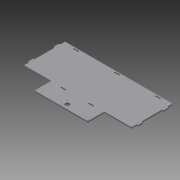
# Autodesk Inventor part: FRAME BOTTOM
Saved by Autodesk Inventor 2013 (Build 170138000, 138)
## iProperties
Created: 2014-03-04
Part Number: FRAME BOTTOM
Material: Generic
Document SubType Name: Modeling
Designer: employee
Density: 1 g/cm^3
Author: employee
Autodesk Inventor part; units mm, degrees
ref_plane "YZ Plane" through (0, 0, 0) normal (1, 0, 0) x (0, 1, 0)
ref_plane "XZ Plane" through (0, 0, 0) normal (0, 1, 0) x (-1, 0, 0)
ref_plane "XY Plane" through (0, 0, 0) normal (0, 0, 1) x (1, 0, 0)
sketch "Sketch1" plane through (0, 0, 0) normal (0, 0, 1) x (1, 0, 0)
  line L0 (-130, -81.477) -> (130, -81.477)
  line L1 (130, -81.477) -> (130, 0)
  line L2 (130, 0) -> (-130, 0)
  line L3 (-130, 0) -> (-130, -81.477)
  line L4 (262.5, 0) -> (-262.5, 0)
  line L5 (-262.5, 0) -> (-262.5, 200)
  line L6 (-262.5, 200) -> (262.5, 200)
  line L7 (262.5, 200) -> (262.5, 0)
  point P0 (0, 0)
  point P1 (0, 0)
  dimension "d0" = 260
  dimension "d2" = 81.477
  dimension "d3" = 525
  dimension "d4" = 200
  constraints: 16 end point, 4 parallel, 2 coincident, 2 horizontal, 2 midpoint, 2 perpendicular
  measures "d0" distance of L1.end L2.end
  measures "d2" distance of L0.end L1.end
  measures "d3" distance of L5.end L6.end
  measures "d4" distance of L4.end L5.end
extrude "Extrusion1" add sketch "Sketch1" along normal blind 6.477
fillet "Fillet1" radius 5 2 edges at (-130, -81.477, 3.2385) (130, -81.477, 3.2385)
sketch "Sketch2" plane through (0, 0, 0) normal (0, 0, -1) x (-1, 0, 0)
  line L0 (-111.6967, -32.977) -> (-111.6967, -8.977) projected
  line L1 (-111.6967, -8.977) -> (-122.3033, -8.977) projected
  line L2 (-122.3033, -8.977) -> (-122.3033, -32.977) projected
  line L3 (-122.3033, -32.977) -> (-111.6967, -32.977) projected
  arc A0 (-109, -81.477) -> (-104, -76.477) centre (-109, -76.477) ccw projected
  line L4 (-109, -81.477) -> (-125, -81.477) projected
  arc A1 (-130, -76.477) -> (-125, -81.477) centre (-125, -76.477) ccw projected
  line L5 (-130, -76.477) -> (-130, -11.477) projected
  arc A2 (-125, -6.477) -> (-130, -11.477) centre (-125, -11.477) ccw projected
  line L6 (-125, -6.477) -> (-109, -6.477) projected
  arc A3 (-104, -11.477) -> (-109, -6.477) centre (-109, -11.477) ccw projected
  line L7 (-104, -11.477) -> (-104, -76.477) projected
  line L8 (-111.6967, -54.977) -> (-122.3033, -54.977) projected
  line L9 (-122.3033, -54.977) -> (-122.3033, -78.977) projected
  line L10 (-122.3033, -78.977) -> (-111.6967, -78.977) projected
  line L11 (-111.6967, -78.977) -> (-111.6967, -54.977) projected
  line L12 (-108, -29.977) -> (-108, -25.977) projected
  line L13 (-108, -25.977) -> (-109.5, -25.977) projected
  line L14 (-109.5, -25.977) -> (-109.5, -29.977) projected
  line L15 (-109.5, -29.977) -> (-108, -29.977) projected
  line L16 (-124.5, -29.977) -> (-124.5, -25.977) projected
  line L17 (-124.5, -25.977) -> (-126, -25.977) projected
  line L18 (-126, -25.977) -> (-126, -29.977) projected
  line L19 (-126, -29.977) -> (-124.5, -29.977) projected
  line L20 (-109.5, -11.977) -> (-109.5, -15.977) projected
  line L21 (-109.5, -15.977) -> (-108, -15.977) projected
  line L22 (-108, -15.977) -> (-108, -11.977) projected
  line L23 (-108, -11.977) -> (-109.5, -11.977) projected
  line L24 (-126, -11.977) -> (-126, -15.977) projected
  line L25 (-126, -15.977) -> (-124.5, -15.977) projected
  line L26 (-124.5, -15.977) -> (-124.5, -11.977) projected
  line L27 (-124.5, -11.977) -> (-126, -11.977) projected
  line L28 (-124.5, -75.977) -> (-124.5, -71.977) projected
  line L29 (-124.5, -71.977) -> (-126, -71.977) projected
  line L30 (-126, -71.977) -> (-126, -75.977) projected
  line L31 (-126, -75.977) -> (-124.5, -75.977) projected
  line L32 (-108, -57.977) -> (-109.5, -57.977) projected
  line L33 (-109.5, -57.977) -> (-109.5, -61.977) projected
  line L34 (-109.5, -61.977) -> (-108, -61.977) projected
  line L35 (-108, -61.977) -> (-108, -57.977) projected
  line L36 (-126, -57.977) -> (-126, -61.977) projected
  line L37 (-126, -61.977) -> (-124.5, -61.977) projected
  line L38 (-124.5, -61.977) -> (-124.5, -57.977) projected
  line L39 (-124.5, -57.977) -> (-126, -57.977) projected
  line L40 (-109.5, -75.977) -> (-108, -75.977) projected
  line L41 (-108, -75.977) -> (-108, -71.977) projected
  line L42 (-108, -71.977) -> (-109.5, -71.977) projected
  line L43 (-109.5, -71.977) -> (-109.5, -75.977) projected
  line L44 (122.3033, -32.977) -> (122.3033, -8.977) projected
  line L45 (122.3033, -8.977) -> (111.6967, -8.977) projected
  line L46 (111.6967, -8.977) -> (111.6967, -32.977) projected
  line L47 (111.6967, -32.977) -> (122.3033, -32.977) projected
  arc A4 (125, -81.477) -> (130, -76.477) centre (125, -76.477) ccw projected
  line L48 (125, -81.477) -> (109, -81.477) projected
  arc A5 (104, -76.477) -> (109, -81.477) centre (109, -76.477) ccw projected
  line L49 (104, -76.477) -> (104, -11.477) projected
  arc A6 (109, -6.477) -> (104, -11.477) centre (109, -11.477) ccw projected
  line L50 (109, -6.477) -> (125, -6.477) projected
  arc A7 (130, -11.477) -> (125, -6.477) centre (125, -11.477) ccw projected
  line L51 (130, -11.477) -> (130, -76.477) projected
  line L52 (122.3033, -54.977) -> (111.6967, -54.977) projected
  line L53 (111.6967, -54.977) -> (111.6967, -78.977) projected
  line L54 (111.6967, -78.977) -> (122.3033, -78.977) projected
  line L55 (122.3033, -78.977) -> (122.3033, -54.977) projected
  line L56 (126, -29.977) -> (126, -25.977) projected
  line L57 (126, -25.977) -> (124.5, -25.977) projected
  line L58 (124.5, -25.977) -> (124.5, -29.977) projected
  line L59 (124.5, -29.977) -> (126, -29.977) projected
  line L60 (109.5, -29.977) -> (109.5, -25.977) projected
  line L61 (109.5, -25.977) -> (108, -25.977) projected
  line L62 (108, -25.977) -> (108, -29.977) projected
  line L63 (108, -29.977) -> (109.5, -29.977) projected
  line L64 (124.5, -11.977) -> (124.5, -15.977) projected
  line L65 (124.5, -15.977) -> (126, -15.977) projected
  line L66 (126, -15.977) -> (126, -11.977) projected
  line L67 (126, -11.977) -> (124.5, -11.977) projected
  line L68 (108, -11.977) -> (108, -15.977) projected
  line L69 (108, -15.977) -> (109.5, -15.977) projected
  line L70 (109.5, -15.977) -> (109.5, -11.977) projected
  line L71 (109.5, -11.977) -> (108, -11.977) projected
  line L72 (109.5, -75.977) -> (109.5, -71.977) projected
  line L73 (109.5, -71.977) -> (108, -71.977) projected
  line L74 (108, -71.977) -> (108, -75.977) projected
  line L75 (108, -75.977) -> (109.5, -75.977) projected
  line L76 (126, -57.977) -> (124.5, -57.977) projected
  line L77 (124.5, -57.977) -> (124.5, -61.977) projected
  line L78 (124.5, -61.977) -> (126, -61.977) projected
  line L79 (126, -61.977) -> (126, -57.977) projected
  line L80 (108, -57.977) -> (108, -61.977) projected
  line L81 (108, -61.977) -> (109.5, -61.977) projected
  line L82 (109.5, -61.977) -> (109.5, -57.977) projected
  line L83 (109.5, -57.977) -> (108, -57.977) projected
  line L84 (124.5, -75.977) -> (126, -75.977) projected
  line L85 (126, -75.977) -> (126, -71.977) projected
  line L86 (126, -71.977) -> (124.5, -71.977) projected
  line L87 (124.5, -71.977) -> (124.5, -75.977) projected
  point P0 (0, 0)
extrude "Extrusion2" cut sketch "Sketch2" against normal through all contours L15 L14 L13 L12 | L19 L18 L17 L16 | L23 L22 L21 L20 | L27 L26 L25 L24 | L31 L30 L29 L28 | L35 L34 L33 L32 | L39 L38 L37 L36 | L43 L42 L41 L40 | L59 L58 L57 L56 | L63 L62 L61 L60 | L67 L66 L65 L64 | L71 L70 L69 L68 | L75 L74 L73 L72 | L79 L78 L77 L76 | L83 L82 L81 L80 | L87 L86 L85 L84
sketch "Sketch3" plane through (0, 0, 0) normal (0, 0, -1) x (-1, 0, 0)
  line L0 (125, -81.477) -> (-125, -81.477) projected
  line L1 (11.5, -81.477) -> (-30.5, -81.477)
  line L2 (-30.5, -81.477) -> (-30.5, -39.477)
  line L3 (-30.5, -39.477) -> (11.5, -39.477)
  line L4 (11.5, -39.477) -> (11.5, -81.477)
  circle A0 centre (-9.5, -60.477) radius 11
  line L5 (-25, -44.977) -> (6, -44.977)
  line L6 (6, -44.977) -> (6, -75.977)
  line L7 (6, -75.977) -> (-25, -75.977)
  line L8 (-25, -75.977) -> (-25, -44.977)
  circle A1 centre (-25, -75.977) radius 1.5
  circle A2 centre (6, -75.977) radius 1.5
  circle A3 centre (6, -44.977) radius 1.5
  circle A4 centre (-25, -44.977) radius 1.5
  point P0 (0, 0)
  point P1 (-9.5, -39.477)
  point P2 (11.5, -60.477)
  dimension "d10" = 9.5
  dimension "d11" = 42
  dimension "d12" = 22
  dimension "d13" = 31
  dimension "d14" = 3
  constraints: 16 end point, 5 centre point, 5 coincident, 3 equal radius, 2 horizontal, 2 midpoint, 2 parallel, 2 perpendicular, 1 horizontal alignment, 1 point on line, 1 vertical alignment, 9 other
  measures "d10" horizontal distance of point (0, 0) point (-9.5, -39.477)
  measures "d11" distance of L3.end L1.start
  measures "d12" diameter of A0
  measures "d13" distance of L6.end L7.end
  measures "d14" diameter of A1
extrude "Extrusion3" cut sketch "Sketch3" against normal through all contours A0 | L8 A4 L5 | L5 A4 L8 | A3 L6 L5 | L5 L6 A3 | A1 L7 L8 | L8 L7 A1 | A2 L7 L6 | L6 L7 A2
sketch "Sketch4" plane through (0, 0, 6.477) normal (0, 0, 1) x (1, 0, 0)
  line L0 (262.5, 200) -> (-262.5, 200) projected
  line L1 (-262.5, 200) -> (-262.5, 0) projected
  line L2 (-262.5, 0) -> (-130, 0) projected
  line L3 (-208.75, 0) -> (-183.75, 0)
  line L4 (-183.75, 0) -> (-183.75, -6.477)
  line L5 (-183.75, -6.477) -> (-208.75, -6.477)
  line L6 (-208.75, -6.477) -> (-208.75, 0)
  line L7 (-262.5, 25) -> (-268.977, 25)
  line L8 (-268.977, 25) -> (-268.977, 50)
  line L9 (-268.977, 50) -> (-262.5, 50)
  line L10 (-262.5, 50) -> (-262.5, 25)
  line L11 (-262.5, 175) -> (-268.977, 175)
  line L12 (-268.977, 175) -> (-268.977, 150)
  line L13 (-268.977, 150) -> (-262.5, 150)
  line L14 (-262.5, 150) -> (-262.5, 175)
  point P0 (0, 0)
  point P1 (-196.25, 0)
  point P2 (-196.25, 0)
  dimension "d17" = 25
  dimension "d18" = 25
  dimension "d19" = 25
  dimension "d20" = 6.477
  constraints: 24 end point, 6 parallel, 4 equal length, 3 horizontal, 3 perpendicular, 3 point on line, 2 midpoint, 1 coincident
  measures "d17" distance between parallel lines of L7 L2
  measures "d18" distance between parallel lines of L0 L11
  measures "d19" distance of L4.end L5.end
  measures "d20" distance of L5.end L3.start
extrude "Extrusion4" add sketch "Sketch4" against normal up to surface (6.477 mm away) contours L1 L7 L8 L9 | L1 L13 L12 L11
sketch "Sketch5" plane through (0, 0, 6.477) normal (0, 0, 1) x (1, 0, 0)
  line L0 (-268.977, 175) -> (-268.977, 150) projected
  line L1 (-268.977, 50) -> (-268.977, 25) projected
  line L2 (-260, 164.5) -> (-258.5, 164.5)
  line L3 (-258.5, 164.5) -> (-258.5, 160.5)
  line L4 (-258.5, 160.5) -> (-260, 160.5)
  line L5 (-260, 160.5) -> (-260, 164.5)
  line L6 (-260, 39.5) -> (-258.5, 39.5)
  line L7 (-258.5, 39.5) -> (-258.5, 35.5)
  line L8 (-258.5, 35.5) -> (-260, 35.5)
  line L9 (-260, 35.5) -> (-260, 39.5)
  point P0 (-262.5, 150)
  point P1 (0, 0)
  point P2 (-268.977, 37.5)
  point P3 (-260, 37.5)
  point P4 (-268.977, 162.5)
  point P5 (-260, 162.5)
  dimension "d23" = 2.5
  dimension "d24" = 4
  dimension "d25" = 1.5
  constraints: 16 end point, 4 midpoint, 4 parallel, 2 equal length, 2 horizontal, 2 horizontal alignment, 2 perpendicular, 1 vertical alignment
  measures "d23" horizontal distance of L4.end point (-262.5, 150)
  measures "d24" distance of L2.end L3.end
  measures "d25" distance of L2.start L2.end
extrude "Extrusion5" cut sketch "Sketch5" against normal through all
mirror "Mirror2" about plane through (0, 0, 0) normal (1, 0, 0) of "Extrusion4", "Extrusion5"
sketch "Sketch6" plane through (0, 0, 6.477) normal (0, 0, 1) x (1, 0, 0)
  line L0 (-187.5, 195) -> (-212.5, 195) projected
  line L1 (-187.5, 195) -> (-212.5, 195) projected
  line L2 (-212.5, 195) -> (-212.5, 188.523) projected
  line L3 (-187.5, 188.523) -> (-212.5, 188.523) projected
  line L4 (-187.5, 195) -> (-187.5, 188.523) projected
  line L5 (12.5, 195) -> (-12.5, 195) projected
  line L6 (-12.5, 195) -> (-12.5, 188.523) projected
  line L7 (12.5, 188.523) -> (-12.5, 188.523) projected
  line L8 (12.5, 195) -> (12.5, 188.523) projected
  line L9 (187.5, 195) -> (212.5, 195) projected
  line L10 (187.5, 195) -> (187.5, 188.523) projected
  line L11 (187.5, 188.523) -> (212.5, 188.523) projected
  line L12 (212.5, 195) -> (212.5, 188.523) projected
  line L13 (80, 0) -> (55, 0) projected
  line L14 (55, -6.477) -> (55, 0) projected
  line L15 (55, -6.477) -> (80, -6.477) projected
  line L16 (80, -6.477) -> (80, 0) projected
  line L17 (-80, 0) -> (-55, 0) projected
  line L18 (-80, -6.477) -> (-80, 0) projected
  line L19 (-55, -6.477) -> (-80, -6.477) projected
  line L20 (-55, -6.477) -> (-55, 0) projected
  point P0 (0, 0)
extrude "Extrusion6" cut sketch "Sketch6" against normal through all
sketch "Sketch7" plane through (0, 0, 6.477) normal (0, 0, 1) x (1, 0, 0)
  line L0 (-22.977, -71.477) -> (-22.977, -51.477) projected
  line L1 (-16.5, -71.477) -> (-22.977, -71.477) projected
  line L2 (-16.5, -51.477) -> (-16.5, -71.477) projected
  line L3 (-16.5, -51.477) -> (-22.977, -51.477) projected
  line L4 (35.5, -71.477) -> (35.5, -51.477) projected
  line L5 (41.977, -71.477) -> (35.5, -71.477) projected
  line L6 (41.977, -51.477) -> (41.977, -71.477) projected
  line L7 (41.977, -51.477) -> (35.5, -51.477) projected
  point P0 (0, 0)
extrude "Extrusion7" cut sketch "Sketch7" against normal through all
sketch "Sketch8" plane through (0, 0, 6.477) normal (0, 0, 1) x (1, 0, 0)
  line L0 (-22.977, -71.477) -> (-22.977, -51.477) projected
  line L1 (-22.977, -51.477) -> (-16.5, -51.477) projected
  line L2 (-80, -6.477) -> (-80, 0) projected
  line L3 (-80, 0) -> (-55, 0) projected
  line L4 (-55, -6.477) -> (-80, -6.477) projected
  line L5 (-26.977, -59.477) -> (-25.477, -59.477)
  line L6 (-25.477, -59.477) -> (-25.477, -63.477)
  line L7 (-25.477, -63.477) -> (-26.977, -63.477)
  line L8 (-26.977, -63.477) -> (-26.977, -59.477)
  line L9 (-25.477, -63.477) -> (-14, -63.477)
  line L10 (-14, -63.477) -> (-14, -59.477)
  line L11 (-14, -59.477) -> (-25.477, -59.477)
  line L12 (-25.477, -59.477) -> (-25.477, -63.477)
  line L13 (-14, -59.477) -> (-12.5, -59.477)
  line L14 (-12.5, -59.477) -> (-12.5, -63.477)
  line L15 (-12.5, -63.477) -> (-14, -63.477)
  line L16 (-14, -63.477) -> (-14, -59.477)
  line L17 (31.5, -59.477) -> (33, -59.477)
  line L18 (33, -59.477) -> (33, -63.477)
  line L19 (33, -63.477) -> (31.5, -63.477)
  line L20 (31.5, -63.477) -> (31.5, -59.477)
  line L21 (33, -63.477) -> (44.477, -63.477)
  line L22 (44.477, -63.477) -> (44.477, -59.477)
  line L23 (44.477, -59.477) -> (33, -59.477)
  line L24 (33, -59.477) -> (33, -63.477)
  line L25 (44.477, -59.477) -> (45.977, -59.477)
  line L26 (45.977, -59.477) -> (45.977, -63.477)
  line L27 (45.977, -63.477) -> (44.477, -63.477)
  line L28 (44.477, -63.477) -> (44.477, -59.477)
  line L29 (-69.5, 2.5) -> (-65.5, 2.5)
  line L30 (-65.5, 2.5) -> (-65.5, -8.977) construction
  line L31 (-65.5, -8.977) -> (-69.5, -8.977)
  line L32 (-69.5, -8.977) -> (-69.5, 2.5)
  line L33 (-69.5, -8.977) -> (-65.5, -8.977)
  line L34 (-65.5, -8.977) -> (-65.5, -10.477)
  line L35 (-65.5, -10.477) -> (-69.5, -10.477)
  line L36 (-69.5, -10.477) -> (-69.5, -8.977)
  line L37 (-69.5, 2.5) -> (-65.5, 2.5)
  line L38 (-65.5, 2.5) -> (-65.5, 4)
  line L39 (-65.5, 4) -> (-69.5, 4)
  line L40 (-69.5, 4) -> (-69.5, 2.5)
  line L41 (65.5, 2.5) -> (69.5, 2.5)
  line L42 (69.5, 2.5) -> (69.5, -8.977) construction
  line L43 (69.5, -8.977) -> (65.5, -8.977)
  line L44 (65.5, -8.977) -> (65.5, 2.5)
  line L45 (65.5, -8.977) -> (69.5, -8.977)
  line L46 (69.5, -8.977) -> (69.5, -10.477)
  line L47 (69.5, -10.477) -> (65.5, -10.477)
  line L48 (65.5, -10.477) -> (65.5, -8.977)
  line L49 (65.5, 2.5) -> (69.5, 2.5)
  line L50 (69.5, 2.5) -> (69.5, 4)
  line L51 (69.5, 4) -> (65.5, 4)
  line L52 (65.5, 4) -> (65.5, 2.5)
  line L53 (198, 197.5) -> (202, 197.5)
  line L54 (202, 197.5) -> (202, 186.023) construction
  line L55 (202, 186.023) -> (198, 186.023)
  line L56 (198, 186.023) -> (198, 197.5)
  line L57 (198, 186.023) -> (202, 186.023)
  line L58 (202, 186.023) -> (202, 184.523)
  line L59 (202, 184.523) -> (198, 184.523)
  line L60 (198, 184.523) -> (198, 186.023)
  line L61 (198, 197.5) -> (202, 197.5)
  line L62 (202, 197.5) -> (202, 199)
  line L63 (202, 199) -> (198, 199)
  line L64 (198, 199) -> (198, 197.5)
  line L65 (-2, 197.5) -> (2, 197.5)
  line L66 (2, 197.5) -> (2, 186.023) construction
  line L67 (2, 186.023) -> (-2, 186.023)
  line L68 (-2, 186.023) -> (-2, 197.5)
  line L69 (-2, 186.023) -> (2, 186.023)
  line L70 (2, 186.023) -> (2, 184.523)
  line L71 (2, 184.523) -> (-2, 184.523)
  line L72 (-2, 184.523) -> (-2, 186.023)
  line L73 (-2, 197.5) -> (2, 197.5)
  line L74 (2, 197.5) -> (2, 199)
  line L75 (2, 199) -> (-2, 199)
  line L76 (-2, 199) -> (-2, 197.5)
  line L77 (-202, 197.5) -> (-198, 197.5)
  line L78 (-198, 197.5) -> (-198, 186.023) construction
  line L79 (-198, 186.023) -> (-202, 186.023)
  line L80 (-202, 186.023) -> (-202, 197.5)
  line L81 (-202, 186.023) -> (-198, 186.023)
  line L82 (-198, 186.023) -> (-198, 184.523)
  line L83 (-198, 184.523) -> (-202, 184.523)
  line L84 (-202, 184.523) -> (-202, 186.023)
  line L85 (-202, 197.5) -> (-198, 197.5)
  line L86 (-198, 197.5) -> (-198, 199)
  line L87 (-198, 199) -> (-202, 199)
  line L88 (-202, 199) -> (-202, 197.5)
  point P0 (0, 0)
  point P1 (-19.7385, -59.477)
  point P2 (-19.7385, -51.477)
  point P3 (-25.477, -61.477)
  point P4 (-22.977, -61.477)
  point P5 (38.7385, -59.477)
  point P6 (33, -61.477)
  point P7 (35.5, -61.477)
  point P8 (-67.5, 2.5)
  point P9 (-67.5, 0)
  point P10 (-80, -3.2385)
  point P11 (-69.5, -3.2385)
  point P12 (67.5, 2.5)
  point P13 (67.5, 0)
  point P14 (65.5, -3.2385)
  point P15 (200, 197.5)
  point P16 (200, 195)
  point P17 (198, 191.7615)
  point P18 (0, 197.5)
  point P19 (0, 195)
  point P20 (-2, 191.7615)
  point P21 (-200, 197.5)
  point P22 (-200, 195)
  point P23 (-202, 191.7615)
  dimension "d33" = 2.5
  dimension "d34" = 1.5
  dimension "d35" = 4
  dimension "d36" = 1.5
  dimension "d37" = 4
  dimension "d38" = 2.5
  dimension "d39" = 1.5
  dimension "d40" = 4
  dimension "d41" = 1.5
  dimension "d42" = 4
  dimension "d43" = 1.5
  dimension "d44" = 4
  dimension "d45" = 1.5
  dimension "d46" = 4
  dimension "d47" = 1.5
  dimension "d48" = 4
  constraints: 168 end point, 42 parallel, 21 horizontal, 21 perpendicular, 18 midpoint, 11 vertical alignment, 7 collinear, 5 coincident, 5 horizontal alignment
  measures "d33" distance between parallel lines of L0 L12
  measures "d34" distance of L6.end L7.end
  measures "d35" distance of L7.end L5.start
  measures "d36" distance of L21.start L19.end
  measures "d37" distance of L19.end L17.start
  measures "d38" distance from line of L4 L31.end
  measures "d39" distance of L33.end L34.end
  measures "d40" distance of L34.end L35.end
  measures "d41" distance of L45.end L47.start
  measures "d42" distance of L47.start L48.start
  measures "d43" distance of L57.end L59.start
  measures "d44" distance of L59.start L60.start
  measures "d45" distance of L69.end L71.start
  measures "d46" distance of L71.start L72.start
  measures "d47" distance of L81.end L83.start
  measures "d48" distance of L83.start L84.start
extrude "Extrusion8" cut sketch "Sketch8" against normal through all contours L7 L8 L5 L6 | L10 L13 L14 L15 | L40 L39 L38 L29 | L31 L34 L35 L36 | L17 L18 L19 L20 | L25 L26 L27 L22 | L52 L51 L50 L41 | L43 L46 L47 L48 | L64 L63 L62 L53 | L55 L58 L59 L60 | L76 L75 L74 L65 | L67 L70 L71 L72 | L88 L87 L86 L77 | L79 L82 L83 L84
sketch "Sketch9" plane through (0, 0, 6.477) normal (0, 0, 1) x (1, 0, 0)
  circle A0 centre (9.5, -60.477) radius 11 projected
  line L0 (5.5, -31.477) -> (7, -31.477)
  line L1 (7, -31.477) -> (7, -35.477)
  line L2 (7, -35.477) -> (5.5, -35.477)
  line L3 (5.5, -35.477) -> (5.5, -31.477)
  line L4 (13.5, -31.477) -> (12, -31.477)
  line L5 (12, -31.477) -> (12, -35.477)
  line L6 (12, -35.477) -> (13.5, -35.477)
  line L7 (13.5, -35.477) -> (13.5, -31.477)
  line L8 (7, -35.477) -> (12, -35.477)
  point P0 (0, 0)
  point P1 (9.5, -35.477)
  dimension "d51" = 2.5
  dimension "d52" = 1.5
  dimension "d53" = 4
  dimension "d54" = 25
  constraints: 18 end point, 4 parallel, 3 horizontal, 2 equal length, 2 perpendicular, 1 midpoint, 1 vertical alignment
  measures "d51" horizontal distance of L1.end A0.centre
  measures "d52" distance of L4.start L4.end
  measures "d53" distance of L6.end L4.start
  measures "d54" distance from line of A0.centre L8
extrude "Extrusion9" cut sketch "Sketch9" against normal through all contours L5 L4 L7 L6 | L0 L1 L2 L3
sketch "Sketch10" plane through (0, 0, 0) normal (0, 0, -1) x (-1, 0, 0)
  circle A0 centre (-170.3448, 131.5769) radius 1.7 construction
  circle A1 centre (-79.6668, 87.7619) radius 1.7 construction
  circle A2 centre (-170.3448, 87.7619) radius 1.7 construction
  circle A3 centre (-79.6668, 131.5769) radius 1.7 construction
  line L0 (-74.2058, 135.0694) -> (-175.8058, 135.0694) construction
  line L1 (-175.8058, 135.0694) -> (-175.8058, 84.2694) construction
  line L2 (-175.8058, 84.2694) -> (-74.2058, 84.2694) construction
  line L3 (-74.2058, 84.2694) -> (-74.2058, 135.0694) construction
  circle A4 centre (66.3099, 91.7331) radius 1.621 construction
  circle A5 centre (216.3099, 141.7331) radius 1.621 construction
  circle A6 centre (216.3099, 91.7331) radius 1.621 construction
  circle A7 centre (66.3099, 141.7331) radius 1.621 construction
  line L4 (248.8099, 59.2331) -> (33.8099, 59.2331) construction
  line L5 (33.8099, 59.2331) -> (33.8099, 174.2331) construction
  line L6 (33.8099, 174.2331) -> (248.8099, 174.2331) construction
  line L7 (248.8099, 174.2331) -> (248.8099, 59.2331) construction
  circle A8 centre (-170.3448, 131.5769) radius 1.5
  circle A9 centre (-170.3448, 87.7619) radius 1.5
  circle A10 centre (-79.6668, 87.7619) radius 1.5
  circle A11 centre (-79.6668, 131.5769) radius 1.5
  circle A12 centre (66.3099, 141.7331) radius 2
  circle A13 centre (66.3099, 91.7331) radius 2
  circle A14 centre (216.3099, 91.7331) radius 2
  circle A15 centre (216.3099, 141.7331) radius 2
  point P0 (0, 0)
  dimension "d57" = 3
  dimension "d59" = 4
  constraints: 8 centre point, 8 coincident, 6 equal radius
  measures "d57" diameter of A9
  measures "d59" diameter of A12
extrude "Extrusion10" cut sketch "Sketch10" against normal blind 4
body "Solid1"
